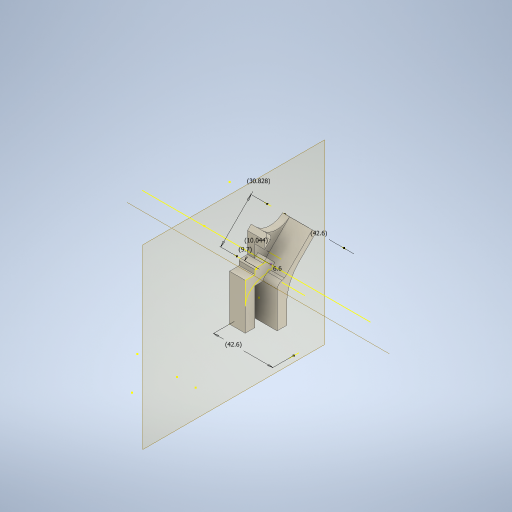
# Autodesk Inventor part: MPM_connector_holder_part_2
Saved by Autodesk Inventor 2023 (Build 270158000, 158)
## iProperties
Created: 2023-06-01
Part Number: MPM_connector_holder_part_2
Material: Generic
Document SubType Name: Modeling
Designer: Daniil
Density: 1 g/cm^3
Appearance: Default
Author: Daniil
Autodesk Inventor part; units mm, degrees
ref_plane "YZ Plane" through (0, 0, 0) normal (1, 0, 0) x (0, 1, 0)
ref_plane "XZ Plane" through (0, 0, 0) normal (0, 1, 0) x (-1, 0, 0)
ref_plane "XY Plane" through (0, 0, 0) normal (0, 0, 1) x (1, 0, 0)
sketch "Sketch1" plane through (0, 0, 0) normal (0, 1, 0) x (-1, 0, 0)
  line L0 (23.4955, 9.8996) -> (-50.8045, 9.8996)
  line L1 (-50.8045, 9.8996) -> (-50.8045, -84.7004)
  line L2 (-50.8045, -84.7004) -> (23.4955, -84.7004)
  line L3 (23.4955, -84.7004) -> (23.4955, 9.8996)
  line L4 (29.4455, 15.7996) -> (-56.7545, 15.7996)
  line L5 (-56.7545, 15.7996) -> (-56.7545, -90.6004)
  line L6 (-56.7545, -90.6004) -> (29.4455, -90.6004)
  line L7 (29.4455, -90.6004) -> (29.4455, 15.7996)
  line L8 (29.4455, -37.4004) -> (-56.7545, -37.4004) construction
  line L9 (-13.6545, -90.6004) -> (-13.6545, 15.7996) construction
  dimension "d0" = 94.6
  dimension "d1" = 74.3
  dimension "d2" = 106.4
  dimension "d3" = 86.2
  constraints: 20 end point, 4 midpoint, 4 parallel, 2 horizontal, 2 perpendicular, 2 other
  measures "d0" distance between parallel lines of L2 L0
  measures "d1" distance between parallel lines of L1 L3
  measures "d2" distance between parallel lines of L6 L4
  measures "d3" distance between parallel lines of L5 L7
extrude "Extrusion1" add sketch "Sketch1" along normal blind 6
fillet "Fillet1" radius 4.5 4 edges at (-23.4955, 3, 9.8996) (50.8045, 3, 9.8996) (50.8045, 3, -84.7004) (-23.4955, 3, -84.7004)
fillet "Fillet2" radius 4.5 4 edges at (56.7545, 3, 15.7996) (-29.4455, 3, 15.7996) (56.7545, 3, -90.6004) (-29.4455, 3, -90.6004)
sketch "Sketch2" plane through (0, 0, 0) normal (0, -1, 0) x (1, 0, 0)
  line L0 (50.8045, -80.2004) -> (50.8045, 5.3996) projected
  arc A0 (46.3045, -84.7004) -> (50.8045, -80.2004) centre (46.3045, -80.2004) ccw projected
  line L1 (-18.9955, -84.7004) -> (46.3045, -84.7004) projected
  arc A1 (-23.4955, -80.2004) -> (-18.9955, -84.7004) centre (-18.9955, -80.2004) ccw projected
  line L2 (-23.4955, 5.3996) -> (-23.4955, -80.2004) projected
  arc A2 (-18.9955, 9.8996) -> (-23.4955, 5.3996) centre (-18.9955, 5.3996) ccw projected
  line L3 (46.3045, 9.8996) -> (-18.9955, 9.8996) projected
  arc A3 (50.8045, 5.3996) -> (46.3045, 9.8996) centre (46.3045, 5.3996) ccw projected
  line L4 (43.8045, -77.7004) -> (-16.4955, -77.7004)
  line L5 (-16.4955, -77.7004) -> (-16.4955, 2.8996)
  line L6 (-16.4955, 2.8996) -> (43.8045, 2.8996)
  line L7 (43.8045, 2.8996) -> (43.8045, -77.7004)
  line L8 (13.6545, -84.7004) -> (13.6545, 9.8996) construction
  line L9 (46.3045, 9.8996) -> (-18.9955, 9.8996) construction
  line L10 (50.8045, -80.2004) -> (50.8045, 5.3996) construction
  line L11 (50.8045, -37.4004) -> (-23.4955, -37.4004) construction
  line L12 (56.7545, 11.2996) -> (56.7545, -86.1004) construction
  point P0 (0, 0)
  dimension "d8" = 5.95
  dimension "d9" = 7
  dimension "d10" = 7
  constraints: 12 end point, 4 midpoint, 2 parallel, 1 horizontal, 1 perpendicular, 2 other
  measures "d8" distance between parallel lines of L0 L12
  measures "d9" distance between parallel lines of L7 L0
  measures "d10" distance between parallel lines of L1 L4
extrude "Extrusion2" add sketch "Sketch2" along normal blind 6
fillet "Fillet3" radius 4.5 4 edges at (43.8045, -3, -77.7004) (43.8045, -3, 2.8996) (-16.4955, -3, 2.8996) (-16.4955, -3, -77.7004)
sketch "Sketch3" plane through (0, 0, 0) normal (0, 1, 0) x (1, 0, 0)
  arc A0 (46.3045, -9.8996) -> (50.8045, -5.3996) centre (46.3045, -5.3996) ccw projected
  line L0 (50.8045, 80.2004) -> (50.8045, -5.3996) projected
  arc A1 (50.8045, 80.2004) -> (46.3045, 84.7004) centre (46.3045, 80.2004) ccw projected
  line L1 (-18.9955, 84.7004) -> (46.3045, 84.7004) projected
  arc A2 (-18.9955, 84.7004) -> (-23.4955, 80.2004) centre (-18.9955, 80.2004) ccw projected
  line L2 (-23.4955, -5.3996) -> (-23.4955, 80.2004) projected
  arc A3 (-23.4955, -5.3996) -> (-18.9955, -9.8996) centre (-18.9955, -5.3996) ccw projected
  line L3 (46.3045, -9.8996) -> (-18.9955, -9.8996) projected
  arc A4 (43.8045, 73.2004) -> (39.3045, 77.7004) centre (39.3045, 73.2004) ccw projected
  line L4 (43.8045, 1.6004) -> (43.8045, 73.2004) projected
  arc A5 (39.3045, -2.8996) -> (43.8045, 1.6004) centre (39.3045, 1.6004) ccw projected
  line L5 (-11.9955, -2.8996) -> (39.3045, -2.8996) projected
  arc A6 (-16.4955, 1.6004) -> (-11.9955, -2.8996) centre (-11.9955, 1.6004) ccw projected
  line L6 (-16.4955, 73.2004) -> (-16.4955, 1.6004) projected
  arc A7 (-11.9955, 77.7004) -> (-16.4955, 73.2004) centre (-11.9955, 73.2004) ccw projected
  line L7 (39.3045, 77.7004) -> (-11.9955, 77.7004) projected
  point P0 (0, 0)
extrude "Extrusion3" add sketch "Sketch3" along normal blind 2
ref_plane "Work Plane1" through (-23.4955, 6, -84.7004) normal (0, 0.7071068, -0.7071068) x (1, 0, 0)
sketch "Sketch5" plane through (-23.4955, 6, -84.7004) normal (0, 0.7071068, -0.7071068) x (1, 0, 0)
  line L0 (4.5, 0) -> (69.8, 0) projected
  line L1 (37.15, 0) -> (37.15, -42.3796) construction
  circle A0 centre (37.15, 1.34) radius 1.34 construction
  line L2 (37.15, 1.34) -> (37.15, -18.66) construction
  line L3 (38.49, 1.34) -> (38.49, -18.66)
  line L4 (35.81, -18.66) -> (35.81, 1.34)
  arc A1 (38.49, 1.34) -> (35.81, 1.34) centre (37.15, 1.34) ccw
  arc A2 (35.81, -18.66) -> (38.49, -18.66) centre (37.15, -18.66) ccw
  point P0 (23.4955, -55.6496)
  point P1 (37.15, -8.66)
  dimension "d20" = 2.68
  dimension "d19" = 90
  dimension "d21" = 20
  dimension "d22" = 2.68
  constraints: 10 end point, 4 point on circle, 4 tangent, 2 centre point, 2 midpoint, 1 horizontal, 1 parallel, 1 point on line, 1 vertical, 1 vertical alignment, 2 other
  measures "d19" angle of L0 L1
  measures "d21" distance of L2.start L2.end
  measures "d22" distance between parallel lines of L4 L3
extrude "Extrusion5" cut sketch "Sketch5" along normal mid plane 51.82
sketch "Sketch6" plane through (-23.4955, 6, -84.7004) normal (0, 0.7071068, -0.7071068) x (1, 0, 0)
  arc A0 (38.49, 1.34) -> (35.81, 1.34) centre (37.15, 1.34) ccw projected
  line L0 (38.49, 0) -> (38.49, 1.34) projected
  arc A1 (38.49, 1.34) -> (35.81, 1.34) centre (37.15, 1.34) ccw projected
  line L1 (35.81, 1.34) -> (35.81, 0) projected
  line L2 (4.5, 0) -> (35.81, 0) projected
  line L3 (4.5, 2.8284) -> (4.5, 0) projected
  line L4 (4.5, 2.8284) -> (69.8, 2.8284) projected
  line L5 (69.8, 0) -> (69.8, 2.8284) projected
  line L6 (38.49, 0) -> (69.8, 0) projected
  line L7 (75.75, 8.4146) -> (-1.45, 8.4146) projected
  line L8 (74.9473, 2.68) -> (-18.0058, 2.68) construction
  line L9 (0, -55.225) -> (0, 5.3033) construction
  line L10 (90.8097, 9.1284) -> (-67.1811, 9.1284) construction
  line L11 (37.15, 2.68) -> (37.15, 37.6448) construction
  line L12 (58.45, 9.1284) -> (15.85, 9.1284)
  line L13 (15.85, 9.1284) -> (15.85, 13.1284)
  line L14 (15.85, 13.1284) -> (58.45, 13.1284)
  line L15 (58.45, 13.1284) -> (58.45, 9.1284)
  point P0 (23.4955, -55.6496)
  dimension "d25" = 6.3
  dimension "d26" = 42.6
  dimension "d27" = 4
  constraints: 14 end point, 3 perpendicular, 2 horizontal, 2 parallel, 2 point on line, 1 point on circle, 1 tangent, 1 other
  measures "d25" distance between parallel lines of L10 L4
  measures "d26" distance between parallel lines of L13 L15
  measures "d27" distance between parallel lines of L14 L10
extrude "Extrusion6" add sketch "Sketch6" along normal blind 35 contours L12 L13 L14 L15
sketch "Sketch7" plane through (-23.4955, 30.7487, -109.4492) normal (0, 0.7071068, -0.7071068) x (-1, 0, 0)
  line L0 (-15.85, -13.1284) -> (-15.85, -9.1284) projected
  line L1 (-58.45, -9.1284) -> (-58.45, -13.1284) projected
  point P0 (-23.4955, 55.6496)
  point P1 (-15.85, -11.1284)
  point P2 (-58.45, -11.1284)
  dimension "d30" = 42.6
  constraints: 2 midpoint
  measures "d30" distance of point (-15.85, -11.128) point (-58.45, -11.128)
sketch "Sketch8" plane through (34.9545, -3.2832, -93.9836) normal (1, 0, 0) x (0, 0.7071068, -0.7071068)
  line L0 (-0.0707, 4.7139) -> (-3.2527, 7.8958) projected
  line L1 (0.9899, 12.1385) -> (4.1719, 8.9565) projected
  line L2 (0, 0) -> (35, 0) projected
  line L3 (-0.0707, 4.7139) -> (-14.2134, -9.4288) construction
  line L4 (0, 4) -> (35, 4) projected
  line L5 (0, 4) -> (0, 0) projected
  line L6 (4.1719, 8.9565) -> (-4.7846, 0)
  line L7 (-4.7846, 0) -> (0, 0)
  line L8 (0, 0) -> (0, 4) projected
  line L9 (0, 0) -> (0, 4)
  line L10 (4.1719, 8.9565) -> (4.1719, 4)
  line L11 (0, 4) -> (35, 4) projected
  line L12 (4.1719, 4) -> (0, 4)
  line L13 (-0.0707, 4.7139) -> (4.1719, 8.9565) projected
  point P0 (-64.1349, 68.778)
  point P1 (4.1719, 4)
  constraints: 12 end point, 3 point on line, 2 perpendicular, 1 collinear, 1 horizontal, 1 vertical
extrude "Extrusion7" add sketch "Sketch8" against normal blind 42.6
sketch "Sketch9" plane through (34.9545, -6.6664, -90.6004) normal (1, 0, 0) x (0, 0, -1)
  line L0 (0, 6.6664) -> (0, 0) projected
  line L1 (0, 0) -> (28.1319, 28.1319) projected
  line L2 (0, 0) -> (0, 6.6664) projected
  line L3 (0, 0) -> (0, -20)
  line L4 (0, -20) -> (5, -20)
  line L5 (5, -20) -> (5, 5)
  line L6 (0, 0) -> (28.1319, 28.1319) projected
  line L7 (5, 5) -> (0, 0)
  point P0 (-90.6004, 6.6664)
  point P1 (5, 5)
  dimension "d33" = 5
  dimension "d34" = 20
  constraints: 8 end point, 2 perpendicular, 2 point on line, 1 collinear
  measures "d33" distance between parallel lines of L5 L3
  measures "d34" distance from line of L4 L0.end
extrude "Extrusion8" add sketch "Sketch9" against normal blind 42.6
sketch "Sketch10" plane through (-7.6455, 24.294, -115.9039) normal (0, 0.7071068, 0.7071068) x (1, 0, 0)
  line L0 (0, -30.8281) -> (42.6, -30.8281) projected
  line L1 (42.6, -30.8281) -> (42.6, 0) projected
  line L2 (0, 0) -> (42.6, 0) projected
  line L3 (0, -30.8281) -> (0, 0) projected
  line L4 (42.6, -30.8281) -> (0, -30.8281) projected
  line L5 (0, -30.8281) -> (5, -30.8281)
  line L6 (5, -30.8281) -> (5, 0)
  line L7 (5, 0) -> (0, 0)
  line L8 (0, 0) -> (0, -30.8281)
  line L9 (42.6, 0) -> (0, 0) projected
  line L10 (37.6, 0) -> (42.6, 0)
  line L11 (42.6, 0) -> (42.6, -30.8281)
  line L12 (42.6, -30.8281) -> (37.6, -30.8281)
  line L13 (37.6, -30.8281) -> (37.6, 0)
  point P0 (7.6455, -99.1349)
  point P1 (37.6, 0)
  point P2 (37.6, -30.8281)
  dimension "d37" = 5
  dimension "d38" = 5
  constraints: 16 end point, 4 parallel, 2 horizontal, 2 perpendicular, 2 point on line
  measures "d37" distance between parallel lines of L3 L6
  measures "d38" distance between parallel lines of L1 L13
extrude "Extrusion9" add sketch "Sketch10" along normal blind 19 contours L3 L2 L6 L0 | L13 L2 L1 L0
sketch "Sketch11" plane through (-7.6455, 37.729, -102.4689) normal (0, 0.7071068, 0.7071068) x (1, 0, 0)
  line L0 (0, -30.8281) -> (5, -30.8281) projected
  line L1 (5, 0) -> (0, 0) projected
  point P0 (7.6455, -99.1349)
  point P1 (2.5, 0)
  point P2 (2.5, -30.8281)
  dimension "d41" = 30.8281
  constraints: 2 midpoint
  measures "d41" distance of point (2.5, 0) point (2.5, -30.828)
sketch "Sketch12" plane through (-2.6455, 2.4952, -94.1052) normal (1, 0, 0) x (0, -0.7071068, -0.7071068)
  line L0 (0, 30.8281) -> (0, 0) projected
  line L1 (0, 30.8281) -> (-19, 30.8281) projected
  line L2 (-19, 0) -> (-19, 30.8281) projected
  line L3 (-4.9565, 0) -> (-19, 0) projected
  line L4 (0, 0) -> (-4.9565, 0) projected
  line L5 (-19, 30.8281) -> (-15, 30.8281)
  line L6 (-15, 30.8281) -> (-15, 0)
  line L7 (-15, 0) -> (-19, 0)
  line L8 (-19, 0) -> (-19, 30.8281)
  point P0 (-64.778, -68.3068)
  dimension "d42" = 15
  constraints: 8 end point, 2 parallel, 1 horizontal, 1 perpendicular, 1 point on line
  measures "d42" distance between parallel lines of L0 L6
extrude "Extrusion10" add sketch "Sketch12" along normal blind 8.5 contours L6 L3 L2 L1
sketch "Sketch13" plane through (29.9545, 2.4952, -94.1052) normal (-1, 0, 0) x (0, 0.7071068, 0.7071068)
  line L0 (0, 0) -> (0, 30.8281) projected
  line L1 (4.9565, 0) -> (0, 0) projected
  line L2 (4.9565, 0) -> (19, 0) projected
  line L3 (19, 30.8281) -> (19, 0) projected
  line L4 (0, 30.8281) -> (19, 30.8281) projected
  line L5 (19, 30.8281) -> (7.45, 30.8281)
  line L6 (7.45, 30.8281) -> (7.45, 0)
  line L7 (7.45, 0) -> (19, 0)
  line L8 (19, 0) -> (19, 30.8281)
  point P0 (64.778, -68.3068)
  point P1 (7.45, 30.8281)
  dimension "d45" = 7.45
  constraints: 8 end point, 2 parallel, 1 horizontal, 1 perpendicular, 1 point on line
  measures "d45" distance between parallel lines of L6 L0
extrude "Extrusion11" add sketch "Sketch13" along normal blind 8.5 contours L4 L3 L2 L6
sketch "Sketch14" plane through (34.9545, -26.6664, -90.6004) normal (1, 0, 0) x (0, 0, -1)
  line L0 (5, 25) -> (28.1319, 48.1319) projected
  line L1 (28.1319, 48.1319) -> (11.8685, 64.3954) projected
  line L2 (-9.9303, 42.5967) -> (11.8685, 64.3954) projected
  line L3 (0, 32.6664) -> (-9.9303, 42.5967) projected
  line L4 (0, 26.6664) -> (0, 32.6664) projected
  line L5 (0, 26.6664) -> (0, 0) projected
  line L6 (0, 0) -> (5, 0) projected
  line L7 (5, 0) -> (5, 25) projected
  line L8 (0, 32.6664) -> (3.5048, 29.1616) construction
  line L9 (-9.9303, 42.5967) -> (11.8685, 64.3954) construction
  line L10 (-7.1018, 39.7682) -> (14.6969, 61.567) construction
  line L11 (0, 32.6664) -> (-1.7632, 34.4296) projected
  line L12 (0, 52.5269) -> (0, 32.6664)
  line L13 (-1.7632, 34.4296) -> (-9.9303, 42.5967) projected
  line L14 (0, 32.6664) -> (-9.9303, 42.5967)
  line L15 (-9.9303, 42.5967) -> (0, 52.5269)
  point P0 (-90.6004, 26.6664)
  point P1 (11.8685, 64.3954)
  point P2 (0, 52.5269)
  constraints: 6 end point, 2 collinear, 1 coincident, 1 perpendicular, 1 point on line
extrude "Extrusion12" cut sketch "Sketch14" against normal blind 100 contours L12 L3 L2
sketch "Sketch15" plane through (-23.4955, 30.7487, -109.4492) normal (0, 0.7071068, -0.7071068) x (-1, 0, 0)
  line L0 (-58.45, -13.1284) -> (-15.85, -13.1284) projected
  line L1 (-15.85, -13.1284) -> (-15.85, 9.8716) projected
  line L2 (-15.85, 9.8716) -> (-29.35, 9.8716) projected
  line L3 (-29.35, 5.8716) -> (-29.35, 9.8716) projected
  line L4 (-20.85, 5.8716) -> (-29.35, 5.8716) projected
  line L5 (-20.85, -9.1284) -> (-20.85, 5.8716) projected
  line L6 (-20.85, -9.1284) -> (-53.45, -9.1284) projected
  line L7 (-53.45, -9.1284) -> (-53.45, -1.6784) projected
  line L8 (-53.45, -1.6784) -> (-44.95, -1.6784) projected
  line L9 (-44.95, 9.8716) -> (-44.95, -1.6784) projected
  line L10 (-58.45, 9.8716) -> (-44.95, 9.8716) projected
  line L11 (-58.45, -13.1284) -> (-58.45, 9.8716) projected
  line L12 (-58.45, 9.8716) -> (-44.95, 9.8716)
  line L13 (-44.95, 9.8716) -> (-44.95, 2.3216)
  line L14 (-44.95, 2.3216) -> (-58.45, 2.3216)
  line L15 (-58.45, 2.3216) -> (-58.45, 9.8716)
  point P0 (-23.4955, 55.6496)
  point P1 (-51.7, 2.3216)
  point P2 (-58.45, 2.3216)
  dimension "d52" = 4
  constraints: 8 end point, 2 parallel, 1 horizontal, 1 midpoint, 1 perpendicular, 1 point on line
  measures "d52" distance from line of L8 point (-51.7, 2.322)
extrude "Extrusion13" cut sketch "Sketch15" against normal blind 100 contours L11 L10 L9 L14
sketch "Sketch16" plane through (-2.6455, 24.294, -115.9039) normal (0, 0.7071068, 0.7071068) x (1, 0, 0)
  line L0 (32.6, -30.8281) -> (0, -30.8281) projected
  line L1 (8.5, -20.7846) -> (0, -20.7846) projected
  point P0 (2.6455, -99.1349)
  dimension "d55" = 10.0435
  measures "d55" distance between parallel lines of L1 L0
sketch "Sketch17" plane through (-2.6455, 6, -90.6004) normal (1, 0, 0) x (0, 0, -1)
  line L0 (0, 14.2037) -> (0, 0) projected
  line L1 (3.5048, -3.5048) -> (0, 0) projected
  line L2 (25.3035, 18.294) -> (3.5048, -3.5048) projected
  line L3 (25.3035, 18.294) -> (14.6969, 28.9006) projected
  line L4 (14.6969, 28.9006) -> (0, 14.2037) projected
  line L5 (5.6261, -1.3835) -> (3.5048, -3.5048)
  line L6 (3.5048, -3.5048) -> (0, 0)
  line L7 (0, 0) -> (2.1213, 2.1213)
  line L8 (2.1213, 2.1213) -> (5.6261, -1.3835)
  point P0 (-90.6004, -6)
  dimension "d56" = 3
  constraints: 8 end point, 2 parallel, 1 perpendicular, 1 point on line
  measures "d56" distance between parallel lines of L1 L8
extrude "Extrusion14" add sketch "Sketch17" along normal blind 34.75 contours L7 L8 L2 L1
sketch "Sketch18" plane through (0, -6, 0) normal (0, -1, 0) x (1, 0, 0)
  line L0 (-18.9955, -84.7004) -> (46.3045, -84.7004) projected
  line L1 (39.3045, -77.7004) -> (-11.9955, -77.7004) projected
  line L2 (-7.6455, -95.6004) -> (-7.6455, -90.6004) projected
  line L3 (34.9545, -90.6004) -> (34.9545, -95.6004) projected
  line L4 (-18.9955, -84.7004) -> (46.3045, -84.7004) projected
  line L5 (-7.6455, -84.7004) -> (34.9545, -84.7004)
  line L6 (34.9545, -84.7004) -> (34.9545, -77.7004)
  line L7 (34.9545, -77.7004) -> (-7.6455, -77.7004)
  line L8 (-7.6455, -77.7004) -> (-7.6455, -84.7004)
  point P0 (0, 0)
  constraints: 8 end point, 2 collinear, 2 parallel, 2 point on line, 1 horizontal, 1 perpendicular
extrude "Extrusion15" add sketch "Sketch18" along normal blind 20
fillet "Fillet5" radius 5 2 edges at (5.8545, 36.3148, -103.8831) (21.4545, 30.9761, -109.2218)
sketch "Sketch19" plane through (0, -6, 0) normal (0, -1, 0) x (1, 0, 0)
  line L0 (34.9545, -118.7324) -> (-7.6455, -118.7324) projected
  line L1 (34.9545, -95.6004) -> (34.9545, -118.7324) projected
  line L2 (34.9545, -77.7004) -> (-7.6455, -77.7004) projected
  line L3 (34.9545, -84.7004) -> (34.9545, -77.7004) projected
  line L4 (-7.6455, -77.7004) -> (-7.6455, -84.7004) projected
  line L5 (-7.6455, -95.6004) -> (-7.6455, -118.7324) projected
  line L6 (34.9545, -118.7324) -> (-7.6455, -118.7324)
  line L7 (-7.6455, -118.7324) -> (-7.6455, -77.7004)
  line L8 (-7.6455, -77.7004) -> (34.9545, -77.7004)
  line L9 (34.9545, -77.7004) -> (34.9545, -118.7324)
  point P0 (0, 0)
  point P1 (34.9545, -84.7004)
  point P2 (-7.6455, -84.7004)
  constraints: 8 end point, 2 parallel, 1 horizontal, 1 perpendicular
extrude "Extrusion16" cut sketch "Sketch19" along normal mid plane 100 keep common part
sketch "Sketch20" plane through (34.9545, 2, -77.7004) normal (1, 0, 0) x (0, 0, -1)
  line L0 (7, -28) -> (0, -28) projected
  line L1 (7, -2) -> (7, -28) construction
  line L2 (7, -28) -> (31.0161, -28) construction
  line L3 (17.9, -28.6664) -> (12.9, -28.6664) projected
  line L4 (12.9, -28.6664) -> (17.9, -28.6664)
  line L5 (17.9, -28.6664) -> (17.9, -28)
  line L6 (17.9, -28) -> (12.9, -28)
  line L7 (12.9, -28) -> (12.9, -28.6664)
  point P0 (-77.7004, -2)
  point P1 (17.9, -28.6664)
  constraints: 10 end point, 2 horizontal, 2 parallel, 1 perpendicular, 1 point on line
extrude "Extrusion17" cut sketch "Sketch20" against normal blind 100
sketch "Sketch21" plane through (0, 6, 0) normal (0, 1, 0) x (1, 0, 0)
  line L0 (-7.6455, 84.7004) -> (-7.6455, 90.6004) projected
  line L1 (-7.6455, 84.7004) -> (12.3145, 84.7004) projected
  line L2 (12.3145, 84.7004) -> (12.3145, 86.5955) projected
  ellipse E0 centre (13.6545, 86.5955) end of major axis (13.6545, 88.4905) minor radius 1.34 (14.9945, 86.5955) -> (12.3145, 86.5955) ccw projected
  line L3 (14.9945, 86.5955) -> (14.9945, 84.7004) projected
  line L4 (14.9945, 84.7004) -> (34.9545, 84.7004) projected
  line L5 (34.9545, 90.6004) -> (34.9545, 84.7004) projected
  line L6 (34.9545, 90.6004) -> (29.9545, 90.6004) projected
  line L7 (29.9545, 90.6004) -> (-2.6455, 90.6004) projected
  line L8 (-2.6455, 90.6004) -> (-7.6455, 90.6004) projected
  point P0 (0, 0)
  constraints: 1 other
extrude "Extrusion18" add sketch "Sketch21" along normal blind 5
sketch "Sketch22" plane through (0, 2, 0) normal (0, 1, 0) x (1, 0, 0)
  line L0 (-7.6455, 77.7004) -> (-7.6455, 84.7004) projected
  line L1 (-7.6455, 77.7004) -> (12.3145, 77.7004) projected
  line L2 (12.3145, 77.7004) -> (12.3145, 82.5955) projected
  ellipse E0 centre (13.6545, 82.5955) end of major axis (13.6545, 84.4905) minor radius 1.34 (14.9945, 82.5955) -> (12.3145, 82.5955) ccw projected
  line L3 (14.9945, 82.5955) -> (14.9945, 77.7004) projected
  line L4 (14.9945, 77.7004) -> (34.9545, 77.7004) projected
  line L5 (34.9545, 84.7004) -> (34.9545, 77.7004) projected
  line L6 (-7.6455, 84.7004) -> (34.9545, 84.7004) projected
  point P0 (0, 0)
  constraints: 1 other
extrude "Extrusion19" add sketch "Sketch22" along normal blind 5
sketch "Sketch23" plane through (-23.4955, 6, -84.7004) normal (0, 0.7071068, -0.7071068) x (1, 0, 0)
  arc A0 (38.49, 1.34) -> (35.81, 1.34) centre (37.15, 1.34) ccw projected
  line L0 (37.15, 1.34) -> (37.15, -18.66) construction
  line L1 (35.81, 1.34) -> (35.81, -18.66)
  line L2 (38.49, -18.66) -> (38.49, 1.34)
  arc A1 (38.49, 1.34) -> (35.81, 1.34) centre (37.15, 1.34) ccw
  arc A2 (35.81, -18.66) -> (38.49, -18.66) centre (37.15, -18.66) ccw
  point P0 (23.4955, -55.6496)
  point P1 (37.15, -8.66)
  dimension "d70" = 20
  constraints: 8 end point, 5 tangent, 4 point on circle, 2 centre point, 1 midpoint, 1 parallel, 1 vertical
  measures "d70" distance of L0.start L0.end
extrude "Extrusion20" cut sketch "Sketch23" along normal mid plane 100
sketch "Sketch24" plane through (-2.6455, 11, -90.6004) normal (1, 0, 0) x (0, 0, -1)
  line L0 (2.1213, -2.8787) -> (5.6261, -6.3835) projected
  line L1 (25.3035, 13.294) -> (5.6261, -6.3835) projected
  line L2 (25.3035, 13.294) -> (14.6969, 23.9006) projected
  line L3 (14.6969, 23.9006) -> (0, 9.2037) projected
  line L4 (0, 9.2037) -> (0, 0) projected
  line L5 (0, 0) -> (0, -5) projected
  line L6 (0, -5) -> (2.1213, -2.8787) projected
  line L7 (0, -0.7574) -> (2.1213, -2.8787)
  line L8 (0, -0.7574) -> (0, -5)
  line L9 (0, -11) -> (-5.9, -11) projected
  line L10 (0, -5) -> (2.1213, -2.8787)
  point P0 (-90.6004, -11)
  constraints: 6 end point, 3 perpendicular, 2 point on line
extrude "Extrusion21" add sketch "Sketch24" along normal blind 33.25 contours L6 L5 L7
sketch "Sketch25" plane through (-23.4955, 6, -84.7004) normal (0, 0.7071068, -0.7071068) x (1, 0, 0)
  line L0 (35.81, 1.34) -> (35.81, -5.6569) projected
  line L1 (38.49, -5.6569) -> (38.49, 1.34) projected
  arc A0 (38.49, 1.34) -> (35.81, 1.34) centre (37.15, 1.34) ccw projected
  line L2 (37.15, 1.34) -> (37.15, -8.66) construction
  line L3 (35.81, 1.34) -> (35.81, -8.66)
  line L4 (38.49, -8.66) -> (38.49, 1.34)
  arc A1 (38.49, 1.34) -> (35.81, 1.34) centre (37.15, 1.34) ccw
  arc A2 (35.81, -8.66) -> (38.49, -8.66) centre (37.15, -8.66) ccw
  point P0 (23.4955, -55.6496)
  point P1 (37.15, -3.66)
  dimension "d75" = 10
  constraints: 8 end point, 5 tangent, 4 point on circle, 2 centre point, 1 midpoint, 1 parallel, 1 vertical
  measures "d75" distance of L2.end L2.start
extrude "Extrusion22" cut sketch "Sketch25" along normal mid plane 33.25
fillet "Fillet6" radius 1 2 edges at (2.3345, 11, -84.7004) (24.9745, 11, -84.7004)
fillet "Fillet7" radius 1 8 edges at (12.3145, 10.7071, -84.9933) (12.3145, 8.5, -84.7004) (12.3145, 11, -88.1504) (14.9945, 10.7071, -84.9933) (14.9945, 8.5, -84.7004) (14.9945, 11, -88.1504) (14.9945, 7, -81.2004) (12.3145, 7, -81.2004)
sketch "Sketch26" plane through (-7.6455, 0, -90.6004) normal (-1, 0, 0) x (0, 0, 1)
  line L0 (5.9, 0) -> (5.9, -26) projected
  line L1 (12.9, -26) -> (12.9, 7) projected
  line L2 (-5, -1.6664) -> (-5, -26) projected
  line L3 (0, -26) -> (0, 0) projected
  line L4 (-5, -26) -> (0, -26) projected
  line L5 (-5, -1.6664) -> (-28.1319, 21.4655) projected
  line L6 (-5, -26) -> (-5, -1.6664) projected
  line L7 (-5, -26) -> (-7, -26)
  line L8 (-7, -26) -> (-7, 0.3336)
  line L9 (-5, -1.6664) -> (-28.1319, 21.4655) projected
  line L10 (-7, 0.3336) -> (-5, -1.6664)
  line L11 (-5, -1.6664) -> (-5, -26)
  point P0 (90.6004, 0)
  point P1 (-7, 0.3336)
  dimension "d80" = 7
  dimension "d81" = 5
  dimension "d82" = 2
  constraints: 8 end point, 2 collinear, 1 horizontal, 1 perpendicular, 1 point on line
  measures "d80" distance between parallel lines of L0 L1
  measures "d81" distance between parallel lines of L2 L3
  measures "d82" distance between parallel lines of L8 L2
sketch "Sketch27" plane through (0, -26, 0) normal (0, -1, 0) x (1, 0, 0)
  line L0 (-7.6455, -77.7004) -> (-7.6455, -84.7004) projected
  line L1 (34.9545, -84.7004) -> (34.9545, -77.7004) projected
  point P0 (0, 0)
  point P1 (-7.6455, -81.2004)
  point P2 (34.9545, -81.2004)
  dimension "d83" = 42.6
  constraints: 2 midpoint
  measures "d83" distance of point (-7.645, -81.2) point (34.955, -81.2)
extrude "Extrusion23" add sketch "Sketch26" against normal blind 42.6
fillet "Fillet8" radius 30 1 edges at (13.6545, 0.3336, -97.6004)
ref_plane "Work Plane2" through (13.6545, -2.895, -77.7004) normal (1, 0, 0) x (0, 0, -1)
sketch "Sketch28" plane through (13.6545, -2.895, -77.7004) normal (1, 0, 0) x (0, 0, -1)
  line L0 (45.7087, -33.5387) -> (-16.3366, -33.5387)
  line L1 (-16.3366, -33.5387) -> (-16.3366, 45.9991)
  line L2 (-16.3366, 45.9991) -> (45.7087, 45.9991)
  line L3 (45.7087, 45.9991) -> (45.7087, -33.5387)
  point P0 (-77.7004, 2.895)
  constraints: 8 end point, 2 parallel, 1 horizontal, 1 perpendicular
extrude "Extrusion24" cut sketch "Sketch28" along normal blind 100
sketch "Sketch29" plane through (13.6545, -2.895, -77.7004) normal (1, 0, 0) x (0, 0, -1)
  line L0 (13.0897, 12.948) -> (12.9, 13.1377) projected
  line L1 (12.895, 13.895) -> (12.895, 12.895) projected
  line L2 (13.0897, 12.948) -> (13.9664, 12.0713) projected
  line L3 (13.9664, 12.0713) -> (18.5261, 7.5116) projected
  line L4 (18.5261, 7.5116) -> (38.2035, 27.189) projected
  line L5 (12.9, 23.0987) -> (12.9, 13.895) projected
  line L6 (12.9, 13.1377) -> (18.5261, 7.5116) projected
  line L7 (12.9, 15.9661) -> (12.9, 13.1377)
  line L8 (12.9, 13.1377) -> (18.5261, 7.5116)
  line L9 (18.5261, 7.5116) -> (19.9403, 8.9258)
  line L10 (38.2035, 27.189) -> (18.5261, 7.5116) projected
  line L11 (19.9403, 8.9258) -> (12.9, 15.9661)
  point P0 (-77.7004, 2.895)
  point P1 (19.9403, 8.9258)
  dimension "d92" = 2
  constraints: 8 end point, 2 point on line, 1 collinear, 1 parallel, 1 perpendicular
  measures "d92" distance between parallel lines of L3 L11
extrude "Extrusion25" add sketch "Sketch29" against normal blind 18
sketch "Sketch30" plane through (13.6545, -2.895, -77.7004) normal (1, 0, 0) x (0, 0, -1)
  line L0 (0, -1.895) -> (13.9664, 12.0713) projected
  line L1 (0, -1.895) -> (0, 0) projected
  line L2 (0, -1.895) -> (15.3806, 13.4855)
  line L3 (12.9, 15.9661) -> (12.9, 13.1377) projected
  line L4 (15.3806, 13.4855) -> (12.9, 15.9661)
  line L5 (12.9, 15.9661) -> (0, 15.9661)
  line L6 (0, -23.105) -> (0, -1.895) projected
  line L7 (0, 15.9661) -> (0, -1.895)
  point P0 (-77.7004, 2.895)
  constraints: 8 end point, 2 perpendicular, 1 collinear, 1 point on line
extrude "Extrusion26" cut sketch "Sketch30" against normal blind 10
sketch "Sketch31" plane through (-7.6455, 25.8605, -90.6004) normal (0, 0, 1) x (1, 0, 0)
  line L0 (11.3, -14.8605) -> (11.3, -12.7894) projected
  line L1 (11.3, -12.7894) -> (5, -12.7894) projected
  line L2 (5, -5.6569) -> (5, -12.7894) projected
  line L3 (13.5, -5.6569) -> (5, -5.6569) projected
  line L4 (13.5, 0) -> (13.5, -5.6569) projected
  line L5 (0, 0) -> (13.5, 0) projected
  line L6 (0, -14.8605) -> (0, 0) projected
  line L7 (11.3, -14.8605) -> (0, -14.8605) projected
  line L8 (11.3, -12.7894) -> (5, -12.7894)
  line L9 (5, -12.7894) -> (5, -14.8605)
  line L10 (5, -14.8605) -> (11.3, -14.8605)
  line L11 (11.3, -14.8605) -> (11.3, -12.7894)
  point P0 (7.6455, -25.8605)
  point P1 (5, -12.7894)
  constraints: 8 end point, 2 parallel, 1 horizontal, 1 perpendicular, 1 point on line
extrude "Extrusion27" cut sketch "Sketch31" against normal blind 7 contours L7 L9 L1 L0
sketch "Sketch32" plane through (13.6545, 6.0308, -97.6407) normal (0, 0.7071068, -0.7071068) x (-1, 0, 0)
  line L0 (16.3, 0) -> (16.3, 15) projected
  line L1 (16.3, 0) -> (0, 0) projected
  line L2 (16.3, 0) -> (9.7, 0)
  line L3 (9.7, 0) -> (9.7, 5.4204)
  line L4 (9.7, 5.4204) -> (16.3, 5.4204)
  line L5 (16.3, 5.4204) -> (16.3, 0)
  line L6 (0, -84.75) -> (0, 147.5281) projected
  point P0 (13.6545, 64.778)
  point P1 (9.7, 2.7102)
  dimension "d100" = 6.6
  dimension "d101" = 9.7
  constraints: 8 end point, 2 parallel, 1 horizontal, 1 midpoint, 1 perpendicular
  measures "d100" distance between parallel lines of L0 L3
  measures "d101" distance from line of L6 point (9.7, 2.71)
sketch "Sketch33" plane through (13.6545, -2.895, -77.7004) normal (1, 0, 0) x (0, 0, -1)
  line L0 (0, -1.895) -> (15.3806, 13.4855) projected
  line L1 (79.8676, -51.0015) -> (-84.3778, 113.2439) projected
  line L2 (19.9403, 8.9258) -> (38.2035, 27.189) projected
  line L3 (15.3806, 13.4855) -> (19.9403, 8.9258)
  line L4 (19.9403, 8.9258) -> (18.1725, 7.158)
  line L5 (18.1725, 7.158) -> (13.6128, 11.7178)
  line L6 (13.6128, 11.7178) -> (15.3806, 13.4855)
  point P0 (-77.7004, 2.895)
  point P1 (13.6128, 11.7178)
  dimension "d102" = 2.5
  constraints: 8 end point, 2 parallel, 1 collinear, 1 perpendicular
  measures "d102" distance between parallel lines of L5 L1
extrude "Extrusion28" cut sketch "Sketch33" against normal blind 10
sketch "Sketch34" plane through (13.6545, -2.895, -77.7004) normal (1, 0, 0) x (0, 0, -1)
  line L0 (18.1725, 7.158) -> (13.6128, 11.7178) projected
  line L1 (0, -1.895) -> (13.6128, 11.7178) projected
  line L2 (18.1725, 7.158) -> (13.6128, 11.7178) projected
  line L3 (18.1725, 7.158) -> (38.2035, 27.189) projected
  line L4 (16.7948, 8.5358) -> (14.6735, 6.4145)
  line L5 (13.6128, 11.7178) -> (0, -1.895) projected
  arc A0 (14.6735, 6.4145) -> (3.6254, 1.7304) centre (14.9391, -9.5833) ccw
  line L6 (3.6254, 1.7304) -> (13.6128, 11.7178)
  line L7 (13.6128, 11.7178) -> (16.7948, 8.5358)
  point P0 (-77.7004, 2.895)
  point P1 (3.6254, 1.7304)
  point P2 (16.7948, 8.5358)
  dimension "d105" = 4.5
  dimension "d106" = 3
  dimension "d107" = 16
  constraints: 6 end point, 2 collinear, 2 point on circle, 2 point on line, 2 tangent, 1 centre point, 1 perpendicular
  measures "d105" distance from line of L4.start L1
  measures "d106" distance from line of L4.end L0
  measures "d107" radius of A0
extrude "Extrusion29" cut sketch "Sketch34" against normal blind 10
fillet "Fillet10" radius 10 1 edges at (8.6545, -4.7901, -77.7004)
sketch "Sketch35" plane through (3.6545, -2.895, -77.7004) normal (1, 0, 0) x (0, 0, -1)
  line L0 (14.9711, 13.895) -> (8, 13.895) projected
  arc A0 (8, 13.895) -> (7, 12.895) centre (8, 12.895) ccw projected
  line L1 (7, 9.895) -> (7, 12.895) projected
  line L2 (0, 9.895) -> (7, 9.895) projected
  line L3 (0, -6.0372) -> (0, 9.895) projected
  arc A1 (2.9289, 1.0339) -> (0, -6.0372) centre (10, -6.0372) ccw projected
  line L4 (3.6254, 1.7304) -> (2.9289, 1.0339) projected
  line L5 (14.9711, 13.895) -> (19.9403, 8.9258) projected
  arc A2 (14.6735, 6.4145) -> (3.6254, 1.7304) centre (14.9391, -9.5833) ccw projected
  line L6 (16.7948, 8.5358) -> (14.6735, 6.4145) projected
  line L7 (18.1725, 7.158) -> (16.7948, 8.5358) projected
  line L8 (19.9403, 8.9258) -> (18.1725, 7.158) projected
  point P0 (-77.7004, 2.895)
sketch "Sketch36" plane through (13.6545, -2.895, -77.7004) normal (1, 0, 0) x (0, 0, -1)
  line L0 (38.2035, 27.189) -> (27.5969, 37.7956) projected
  line L1 (41.0319, 24.3606) -> (28.6868, 12.0154) projected
  line L2 (21.2329, 37.0885) -> (12.9, 28.7556) projected
  line L3 (18.1725, 7.158) -> (38.2035, 27.189) projected
  line L4 (41.0319, 24.3606) -> (24.7685, 40.624) projected
  line L5 (24.7685, 40.624) -> (38.2035, 27.189)
  line L6 (38.2035, 27.189) -> (29.0111, 17.9966)
  line L7 (29.0111, 17.9966) -> (15.5761, 31.4317)
  line L8 (15.5761, 31.4317) -> (24.7685, 40.624)
  point P0 (-77.7004, 2.895)
  point P1 (31.486, 33.9065)
  dimension "d111" = 13
  constraints: 8 end point, 2 parallel, 1 collinear, 1 midpoint, 1 perpendicular
  measures "d111" distance from line of point (31.486, 33.907) L7
extrude "Extrusion30" cut sketch "Sketch36" against normal blind 100
sketch "Sketch37" plane through (-7.6455, 37.729, -102.4689) normal (0, 0.7071068, 0.7071068) x (1, 0, 0)
  line L0 (5, -20.7846) -> (5, -27.2925) projected
  line L1 (13.5, -13) -> (13.5, -16.7846) projected
  line L2 (13.5, -16.7846) -> (13.5, -20.7846) projected
  line L3 (13.5, -20.7846) -> (5, -20.7846) projected
  line L4 (5, -13) -> (13.5, -13) projected
  line L5 (13.5, -20.7846) -> (12, -20.7846)
  line L6 (12, -20.7846) -> (12, -13)
  line L7 (12, -13) -> (13.5, -13)
  line L8 (13.5, -13) -> (13.5, -20.7846)
  point P0 (7.6455, -99.1349)
  dimension "d114" = 7
  constraints: 8 end point, 2 parallel, 1 horizontal, 1 perpendicular, 1 point on line
  measures "d114" distance between parallel lines of L6 L0
extrude "Extrusion31" cut sketch "Sketch37" against normal blind 10
fillet "Fillet11" radius 2 1 edges at (4.3545, 27.1224, -94.6907)
fillet "Fillet12" radius 14 1 edges at (-5.1455, 15.1016, -106.7115)
sketch "Sketch38" plane through (3.6545, -2.895, -77.7004) normal (1, 0, 0) x (0, 0, -1)
  line L0 (14.9711, 13.895) -> (8, 13.895) projected
  line L1 (79.8676, -51.0015) -> (-84.3778, 113.2439) projected
  line L2 (18.1725, 7.158) -> (38.2035, 27.189) projected
  line L3 (14.9711, 13.895) -> (19.9403, 8.9258) projected
  line L4 (14.9711, 13.895) -> (17.7995, 13.895)
  line L5 (17.7995, 13.895) -> (21.3545, 10.34)
  line L6 (21.3545, 10.34) -> (19.9403, 8.9258)
  line L7 (19.9403, 8.9258) -> (18.1725, 7.158) projected
  line L8 (19.9403, 8.9258) -> (14.9711, 13.895)
  point P0 (-77.7004, 2.895)
  dimension "d119" = 2
  constraints: 8 end point, 3 point on line, 1 collinear, 1 horizontal, 1 perpendicular
  measures "d119" distance between parallel lines of L1 L5
extrude "Extrusion32" add sketch "Sketch38" against normal blind 10
sketch "Sketch39" plane through (3.6545, -2.895, -77.7004) normal (1, 0, 0) x (0, 0, -1)
  line L0 (17.7995, 13.895) -> (8, 13.895) projected
  arc A0 (8, 13.895) -> (7, 12.895) centre (8, 12.895) ccw projected
  line L1 (7, 9.895) -> (7, 12.895) projected
  line L2 (0, 9.895) -> (7, 9.895) projected
  line L3 (0, -6.0372) -> (0, 9.895) projected
  arc A1 (2.9289, 1.0339) -> (0, -6.0372) centre (10, -6.0372) ccw projected
  line L4 (3.6254, 1.7304) -> (2.9289, 1.0339) projected
  arc A2 (14.6735, 6.4145) -> (3.6254, 1.7304) centre (14.9391, -9.5833) ccw projected
  line L5 (16.7948, 8.5358) -> (14.6735, 6.4145) projected
  line L6 (18.1725, 7.158) -> (16.7948, 8.5358) projected
  line L7 (21.3545, 10.34) -> (18.1725, 7.158) projected
  line L8 (21.3545, 10.34) -> (17.7995, 13.895) projected
  line L9 (17.7995, 13.895) -> (21.3545, 10.34) projected
  line L10 (38.2035, 27.189) -> (21.3545, 10.34) projected
  arc A3 (19.1369, 27.8708) -> (38.2035, 27.189) centre (29.0364, 37.7703) ccw projected
  line L11 (19.1369, 27.8708) -> (18.4045, 28.6032) projected
  line L12 (18.4045, 28.6032) -> (12.9, 23.0987) projected
  line L13 (12.9, 23.0987) -> (12.9, 13.895) projected
  line L14 (12.9, 13.895) -> (17.7995, 13.895) projected
  line L15 (17.7995, 13.895) -> (12.9, 18.7945)
  line L16 (12.9, 18.7945) -> (12.9, 13.895)
  line L17 (12.9, 13.895) -> (17.7995, 13.895)
  point P0 (-77.7004, 2.895)
  point P1 (12.9, 13.895)
  dimension "d122" = 0
  constraints: 6 end point, 2 perpendicular, 1 point on line
  measures "d122" distance between parallel lines of L8 L15
extrude "Extrusion33" add sketch "Sketch39" against normal blind 10 contours L0 L13 L15
sketch "Sketch40" plane through (13.6545, -2.895, -77.7004) normal (1, 0, 0) x (0, 0, -1)
  line L0 (16.7948, 8.5358) -> (14.6735, 6.4145) projected
  line L1 (18.1725, 7.158) -> (16.7948, 8.5358) projected
  line L2 (18.1725, 7.158) -> (38.2035, 27.189) projected
  line L3 (21.3545, 10.34) -> (18.1725, 7.158) projected
  arc A0 (14.6735, 6.4145) -> (18.1725, 7.158) centre (14.5185, 15.7485) ccw
  arc A1 (14.6735, 6.4145) -> (3.6254, 1.7304) centre (14.9391, -9.5833) ccw projected
  point P0 (-77.7004, 2.895)
  constraints: 2 point on circle, 1 centre point, 1 tangent
extrude "Extrusion34" cut sketch "Sketch40" against normal blind 10
sketch "Sketch41" plane through (4.3545, 20.2037, -90.6004) normal (0, -0.7071068, -0.7071068) x (-1, 0, 0)
  arc A0 (2, 7.7846) -> (0, 5.7846) centre (2, 5.7846) ccw projected
  line L0 (0, 5.7846) -> (0, 0) projected
  line L1 (0, 0) -> (7, 0) projected
  line L2 (7, 7.7846) -> (7, 0) projected
  line L3 (7, 7.7846) -> (2, 7.7846) projected
  point P0 (4.3545, -78.3503)
extrude "Extrusion35" add sketch "Sketch41" along normal blind 0.5
sketch "Sketch42" plane through (3.6545, -2.895, -77.7004) normal (1, 0, 0) x (0, 0, -1)
  line L0 (12.9, 18.7945) -> (12.9, 13.895) projected
  line L1 (21.3545, 10.34) -> (12.9, 18.7945) projected
  line L2 (12.9, 13.895) -> (12.9, 28.7556) projected
  line L3 (12.9, 13.895) -> (15.3497, 16.3448)
  line L4 (12.9, 18.7945) -> (21.3545, 10.34) projected
  line L5 (15.3497, 16.3448) -> (12.9, 18.7945)
  line L6 (12.9, 13.895) -> (8, 13.895) projected
  line L7 (12.9, 18.7945) -> (12.9, 13.895)
  point P0 (-77.7004, 2.895)
  constraints: 6 end point, 2 perpendicular, 1 collinear, 1 point on line
extrude "Extrusion36" cut sketch "Sketch42" against normal blind 6.3
sketch "Sketch44" plane through (13.6545, -2.895, -77.7004) normal (1, 0, 0) x (0, 0, -1)
  arc A0 (14.6735, 6.4145) -> (18.1725, 7.158) centre (14.5185, 15.7485) ccw projected
  arc A1 (14.6735, 6.4145) -> (3.6254, 1.7304) centre (14.9391, -9.5833) ccw projected
  line L0 (2.9289, 1.0339) -> (3.6254, 1.7304) projected
  arc A2 (2.9289, 1.0339) -> (0, -6.0372) centre (10, -6.0372) ccw projected
  line L1 (0, -23.105) -> (0, -6.0372) projected
  line L2 (7, -23.105) -> (0, -23.105) projected
  line L3 (7, 2.895) -> (7, -23.105) projected
  line L4 (12.9, 2.895) -> (7, 2.895) projected
  line L5 (12.9, -23.105) -> (12.9, 2.895) projected
  line L6 (19.9, -23.105) -> (12.9, -23.105) projected
  line L7 (19.9, -9.1978) -> (19.9, -23.105) projected
  arc A3 (28.6868, 12.0154) -> (19.9, -9.1978) centre (49.9, -9.1978) ccw projected
  line L8 (41.0319, 24.3606) -> (28.6868, 12.0154) projected
  line L9 (38.2035, 27.189) -> (41.0319, 24.3606) projected
  line L10 (18.1725, 7.158) -> (38.2035, 27.189) projected
  arc A4 (14.6735, 6.4145) -> (18.1725, 7.158) centre (14.5185, 15.7485) ccw projected
  arc A5 (16.459, 6.6171) -> (12.9, 2.895) centre (17.4091, 2.1461) ccw
  point P0 (-77.7004, 2.895)
  constraints: 4 point on circle, 1 centre point, 1 tangent
extrude "Extrusion38" cut sketch "Sketch44" against normal blind 10 contours A0 A5 L4 L3 L2 L1 A2 L0 A1
body "Solid1"
